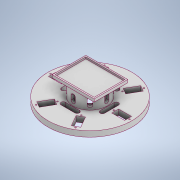
# Autodesk Inventor part: Base
Saved by Autodesk Inventor 2022 (Build 260153000, 153)
## iProperties
Created: 2023-07-22
Part Number: Base
Material: Generic
Document SubType Name: Modeling
Designer: Eric Cao
Density: 1 g/cm^3
Appearance: Pink
Author: Eric Cao
Autodesk Inventor part; units mm, degrees
ref_plane "YZ Plane" through (0, 0, 0) normal (1, 0, 0) x (0, 1, 0)
ref_plane "XZ Plane" through (0, 0, 0) normal (0, 1, 0) x (-1, 0, 0)
sketch "Sketch1" plane through (0, 0, 0) normal (0, 1, 0) x (-1, 0, 0)
  circle A0 centre (0, 0) radius 75
  line L0 (68, 6.15) -> (45, 6.15)
  line L1 (45, 6.15) -> (45, -6.15)
  line L2 (45, -6.15) -> (68, -6.15)
  line L3 (68, -6.15) -> (68, 6.15)
  line L4 (27.8261, 35.8961) -> (39.3261, 55.8147)
  line L5 (28.6739, 61.9647) -> (17.1739, 42.0461)
  line L6 (39.3261, 55.8147) -> (28.6739, 61.9647)
  line L7 (17.1739, 42.0461) -> (27.8261, 35.8961)
  line L8 (-17.1739, 42.0461) -> (-28.6739, 61.9647)
  line L9 (-39.3261, 55.8147) -> (-27.8261, 35.8961)
  line L10 (-28.6739, 61.9647) -> (-39.3261, 55.8147)
  line L11 (-27.8261, 35.8961) -> (-17.1739, 42.0461)
  line L12 (-45, 6.15) -> (-68, 6.15)
  line L13 (-68, -6.15) -> (-45, -6.15)
  line L14 (-68, 6.15) -> (-68, -6.15)
  line L15 (-45, -6.15) -> (-45, 6.15)
  line L16 (-27.8261, -35.8961) -> (-39.3261, -55.8147)
  line L17 (-28.6739, -61.9647) -> (-17.1739, -42.0461)
  line L18 (-39.3261, -55.8147) -> (-28.6739, -61.9647)
  line L19 (-17.1739, -42.0461) -> (-27.8261, -35.8961)
  line L20 (17.1739, -42.0461) -> (28.6739, -61.9647)
  line L21 (39.3261, -55.8147) -> (27.8261, -35.8961)
  line L22 (28.6739, -61.9647) -> (39.3261, -55.8147)
  line L23 (27.8261, -35.8961) -> (17.1739, -42.0461)
  line L24 (0, 0) -> (-29.7165, 0)
  dimension "d7" = 360
  dimension "d54" = 23
  dimension "d55" = 12.3
  dimension "d56" = 45
  constraints: 50 end point, 2 horizontal, 2 parallel, 1 centre point, 1 coincident, 1 perpendicular, 50 other
  measures "d54" distance of L12.start L12.end
  measures "d55" distance of L12.start L13.end
  measures "d56" distance from line of L15 point (0, 0)
extrude "Extrusion1" add sketch "Sketch1" along normal blind 10
sketch "Sketch2" plane through (0, 10, 0) normal (0, 1, 0) x (1, 0, 0)
  line L0 (68, 3.075) -> (68, -9.225)
  circle A0 centre (70.5, 0) radius 1.15
  line L1 (45, 3.075) -> (68, 3.075)
  line L2 (45, -9.225) -> (45, 3.075)
  circle A1 centre (42.5, 0) radius 1.15
  circle A2 centre (35.25, 61.0548) radius 1.15
  circle A3 centre (21.25, 36.8061) radius 1.15
  circle A4 centre (-35.25, 61.0548) radius 1.15
  circle A5 centre (-21.25, 36.8061) radius 1.15
  circle A6 centre (-70.5, 0) radius 1.15
  circle A7 centre (-42.5, 0) radius 1.15
  circle A8 centre (-35.25, -61.0548) radius 1.15
  circle A9 centre (-21.25, -36.8061) radius 1.15
  circle A10 centre (35.25, -61.0548) radius 1.15
  circle A11 centre (21.25, -36.8061) radius 1.15
  point P0 (0, 0)
  dimension "d11" = 2.5
  dimension "d13" = 1.15
  dimension "d14" = 2.5
  dimension "d15" = 1.15
  dimension "d18" = 360
  dimension "d23" = 6.15
  dimension "d24" = 0
  dimension "d58" = 0
  constraints: 12 centre point, 6 end point, 2 coincident, 26 other
  measures "d11" distance from line of L0 point (70.5, 0)
  measures "d13" radius of A0
  measures "d14" distance from line of L2 point (42.5, 0)
  measures "d15" radius of A1
  measures "d23" diameter of A0.centre L1
  measures "d24" vertical distance of A0.centre A1.centre
  measures "d58" distance of point (-70.5, 0) A6.centre
extrude "Extrusion2" cut sketch "Sketch2" against normal blind 4
sketch "Sketch3" plane through (0, 10, 0) normal (0, 1, 0) x (1, 0, 0)
  circle A0 centre (0, 0) radius 15
  dimension "d25" = 30
  constraints: 1 centre point, 1 coincident
  measures "d25" diameter of A0
extrude "Extrusion3" cut sketch "Sketch3" against normal through all
sketch "Sketch4" plane through (0, 10, 0) normal (0, 1, 0) x (1, 0, 0)
  circle A0 centre (0, 0) radius 25
  circle A1 centre (0, 0) radius 30
  line L0 (35, 15.9896) -> (35, -16.9301) construction
  line L1 (31, 11.9896) -> (31, -12.9301)
  line L2 (39, -12.9301) -> (39, 11.9896)
  arc A2 (39, 11.9896) -> (31, 11.9896) centre (35, 11.9896) ccw
  arc A3 (31, -12.9301) -> (39, -12.9301) centre (35, -12.9301) ccw
  arc A4 (12.9301, 31) -> (12.9301, 39) centre (12.9301, 35) ccw
  line L3 (12.9301, 39) -> (-11.9896, 39)
  line L4 (-11.9896, 31) -> (12.9301, 31)
  arc A5 (-11.9896, 39) -> (-11.9896, 31) centre (-11.9896, 35) ccw
  arc A6 (-31, 12.9301) -> (-39, 12.9301) centre (-35, 12.9301) ccw
  line L5 (-39, 12.9301) -> (-39, -11.9896)
  line L6 (-31, -11.9896) -> (-31, 12.9301)
  arc A7 (-39, -11.9896) -> (-31, -11.9896) centre (-35, -11.9896) ccw
  arc A8 (-12.9301, -31) -> (-12.9301, -39) centre (-12.9301, -35) ccw
  line L7 (-12.9301, -39) -> (11.9896, -39)
  line L8 (11.9896, -31) -> (-12.9301, -31)
  arc A9 (11.9896, -39) -> (11.9896, -31) centre (11.9896, -35) ccw
  point P0 (35, -0.4703)
  dimension "d28" = 50
  dimension "d29" = 60
  dimension "d34" = 360
  dimension "d59" = 35
  dimension "d60" = 8
  constraints: 20 end point, 18 point on circle, 10 centre point, 4 tangent, 2 coincident, 2 point on line, 1 midpoint, 1 parallel, 1 vertical, 41 other
  measures "d28" diameter of A0
  measures "d29" diameter of A1
  measures "d59" horizontal distance of point (0, 0) point (35, -0.47)
  measures "d60" distance between parallel lines of L1 L2
extrude "Extrusion4" cut sketch "Sketch4" against normal through all contours A2 L2 A3 L1 | L4 A5 L3 A4 | L6 A7 L5 A6 | L8 A9 L7 A8
extrude "Extrusion5" add sketch "Sketch4" along normal blind 25 contours A1
ref_plane "Work Plane2" through (-30, 10, 0) normal (1, 0, 0) x (0, 0, -1)
sketch "Sketch6" plane through (-30, 10, 0) normal (1, 0, 0) x (0, 0, -1)
  line L0 (0, 18.9497) -> (0, 4.0799) construction
  line L1 (3.6001, 15.3496) -> (3.6001, 7.6799)
  line L2 (-3.6001, 7.6799) -> (-3.6001, 15.3496)
  arc A0 (3.6001, 15.3496) -> (-3.6001, 15.3496) centre (0, 15.3496) ccw
  arc A1 (-3.6001, 7.6799) -> (3.6001, 7.6799) centre (0, 7.6799) ccw
  point P0 (0, -10)
  point P1 (0, 11.5148)
  constraints: 8 end point, 6 point on circle, 4 tangent, 2 centre point, 2 point on line, 1 midpoint, 1 parallel, 1 vertical
extrude "Extrusion6" cut sketch "Sketch6" along normal blind 21.25
pattern_circular "Circular Pattern1" count 8 over 360 about axis through (0, 10, 0) along (0, 1, 0) of "Extrusion6"
sketch "Sketch7" plane through (0, 35, 0) normal (0, 1, 0) x (1, 0, 0)
  line L0 (37.5, 30) -> (-37.5, 30)
  line L1 (-37.5, 30) -> (-37.5, -30)
  line L2 (-37.5, -30) -> (37.5, -30)
  line L3 (37.5, -30) -> (37.5, 30)
  line L4 (0, 0) -> (39.854, 0)
  line L5 (0, 0) -> (0, -35.1958)
  dimension "d45" = 60
  dimension "d46" = 75
  constraints: 12 end point, 2 horizontal, 2 parallel, 1 perpendicular, 1 vertical, 2 other
  measures "d45" distance of L2.end L0.start
  measures "d46" distance between parallel lines of L1 L3
extrude "Extrusion7" add sketch "Sketch7" along normal blind 5
sketch "Sketch8" plane through (0, 40, 0) normal (0, 1, 0) x (1, 0, 0)
  line L0 (35, 27.5) -> (-35, 27.5)
  line L1 (-35, 27.5) -> (-35, -27.5)
  line L2 (-35, -27.5) -> (35, -27.5)
  line L3 (35, -27.5) -> (35, 27.5)
  line L4 (0, 0) -> (53.1918, 0)
  line L5 (0, 0) -> (0, -22.6145)
  dimension "d49" = 55
  dimension "d50" = 70
  constraints: 12 end point, 2 horizontal, 2 parallel, 1 perpendicular, 1 vertical, 2 other
  measures "d49" distance of L2.end L0.start
  measures "d50" distance between parallel lines of L3 L1
extrude "Extrusion8" cut sketch "Sketch8" against normal blind 3
body "Solid1"
